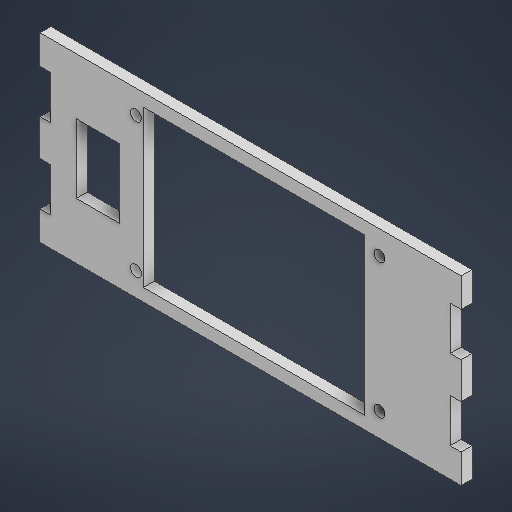
# Autodesk Inventor part: pantallaSoport
Saved by Autodesk Inventor 2026 (Build 300175000, 175)
## iProperties
Created: 2026-04-21
Part Number: pantallaSoport
Material: Generic
Document SubType Name: Modeling
Designer: juana
Density: 1 g/cm^3
Appearance: Default
Author: juana
Autodesk Inventor part; units mm, degrees
ref_plane "YZ Plane" through (0, 0, 0) normal (1, 0, 0) x (0, 1, 0)
ref_plane "XZ Plane" through (0, 0, 0) normal (0, 1, 0) x (-1, 0, 0)
ref_plane "XY Plane" through (0, 0, 0) normal (0, 0, 1) x (1, 0, 0)
sketch "Sketch1" plane through (0, 0, 0) normal (0, 0, 1) x (1, 0, 0)
  line L0 (0, 0) -> (116, 0)
  line L1 (116, 0) -> (116, 50)
  line L2 (116, 50) -> (0, 50)
  line L3 (0, 50) -> (0, 0)
  line L4 (0, 50) -> (3, 50)
  line L5 (3, 50) -> (3, 46.5)
  line L6 (3, 46.5) -> (0, 46.5)
  line L7 (0, 46.5) -> (0, 50)
  line L8 (0, 0) -> (3, 0)
  line L9 (3, 0) -> (3, 3.5)
  line L10 (3, 3.5) -> (0, 3.5)
  line L11 (0, 3.5) -> (0, 0)
  line L12 (58, 0) -> (58, 50) construction
  line L13 (113, 50) -> (113, 46.5)
  line L14 (113, 46.5) -> (116, 46.5)
  line L15 (113, 0) -> (113, 3.5)
  line L16 (113, 3.5) -> (116, 3.5)
  line L17 (19.5, 46.5) -> (96.5, 46.5) construction
  line L18 (96.5, 46.5) -> (96.5, 3.5) construction
  line L19 (96.5, 3.5) -> (19.5, 3.5) construction
  line L20 (19.5, 3.5) -> (19.5, 46.5) construction
  line L21 (28.5, 46.5) -> (89.5, 46.5)
  line L22 (89.5, 46.5) -> (89.5, 3.5)
  line L23 (89.5, 3.5) -> (28.5, 3.5)
  line L24 (28.5, 3.5) -> (28.5, 46.5)
  line L25 (3, 0) -> (0, 0)
  line L26 (0, 0) -> (0, 8)
  line L27 (0, 8) -> (3, 8)
  line L28 (3, 8) -> (3, 0)
  line L29 (0, 50) -> (3, 50)
  line L30 (3, 50) -> (3, 42)
  line L31 (3, 42) -> (0, 42)
  line L32 (0, 42) -> (0, 50)
  line L33 (0, 42) -> (3, 42)
  line L34 (3, 42) -> (3, 30)
  line L35 (3, 30) -> (0, 30)
  line L36 (0, 30) -> (0, 42)
  line L37 (3, 8) -> (0, 8)
  line L38 (0, 8) -> (0, 20)
  line L39 (0, 20) -> (3, 20)
  line L40 (3, 20) -> (3, 8)
  line L41 (116, 8) -> (113, 8)
  line L42 (113, 42) -> (116, 42)
  line L43 (113, 42) -> (113, 30)
  line L44 (113, 30) -> (116, 30)
  line L45 (116, 20) -> (113, 20)
  line L46 (113, 20) -> (113, 8)
  point P0 (1.5, 25)
  point P1 (0, 25)
  point P2 (1.5, 3.5)
  point P3 (19.5, 25)
  point P4 (58, 46.5)
  point P5 (1.5, 46.5)
  point P6 (94.5, 5.5)
  point P7 (94.5, 44.5)
  point P8 (26, 44.5)
  point P9 (26, 5.5)
  point P10 (0, 46.5)
  point P11 (0, 3.5)
  dimension "d0" = 116
  dimension "d1" = 50
  dimension "d2" = 3
  dimension "d4" = 21.5
  dimension "d5" = 21.5
  dimension "d6" = 77
  dimension "d7" = 61
  dimension "d8" = 9
  dimension "d9" = 2
  dimension "d10" = 2
  dimension "d11" = 2
  dimension "d12" = 6.5
  dimension "d13" = 2
  dimension "d34" = 8
  dimension "d35" = 8
  dimension "d36" = 12
  dimension "d37" = 12
  constraints: 94 end point, 18 parallel, 15 symmetric about line, 9 horizontal, 9 perpendicular, 7 midpoint, 7 vertical alignment, 6 horizontal alignment, 2 point on line
  measures "d0" distance of L1.end L2.end
  measures "d1" distance of L0.end L1.end
  measures "d2" distance of L5.end L6.end
  measures "d4" distance from line of L10 point (1.5, 25)
  measures "d5" distance from line of L6 point (1.5, 25)
  measures "d6" distance of L17.start L17.end
  measures "d7" distance of L21.start L21.end
  measures "d8" distance between parallel lines of L20 L24
  measures "d9" distance from line of L19 point (94.5, 5.5)
  measures "d10" distance from line of L17 point (94.5, 44.5)
  measures "d11" distance from line of L18 point (94.5, 44.5)
  measures "d12" distance from line of L20 point (26, 44.5)
  measures "d13" distance from line of L19 point (26, 5.5)
  measures "d34" distance of L27.end L8.end
  measures "d35" distance of L29.end L30.end
  measures "d36" distance of L33.end L34.end
  measures "d37" distance of L39.end L27.end
extrude "Extrusion1" add sketch "Sketch1" along normal blind 3 contours L3 L10 L9 L0 | L9 L28 L40 L39 L3 L35 L34 L30 L5 L2 L13 L14 L1 L42 L43 L44 L45 L46 L41 L16 L15 L0 | L3 L27 L28 L10 | L15 L16 L1 L0 | L3 L6 L30 L31 | L3 L2 L5 L6 | L14 L13 L2 L1
sketch "Sketch2" plane through (0, 0, 3) normal (0, 0, 1) x (1, 0, 0)
  line L0 (28.5, 46.5) -> (89.5, 46.5) projected
  line L1 (19.5, 46.5) -> (96.5, 46.5)
  line L2 (96.5, 46.5) -> (96.5, 3.5)
  line L3 (96.5, 3.5) -> (19.5, 3.5)
  line L4 (19.5, 3.5) -> (19.5, 46.5)
  line L5 (116, 50) -> (0, 50) projected
  line L6 (0, 8) -> (0, 0) projected
  point P0 (26.42, 43.5)
  point P1 (26.42, 6.5)
  point P2 (58, 46.5)
  point P3 (58, 50)
  point P4 (113, 50)
  point P5 (3, 50)
  point P6 (19.5, 25)
  point P7 (0, 25)
  point P8 (0, 46.5)
  point P9 (0, 3.5)
  point P10 (93.5, 43.5)
  point P11 (93.5, 6.5)
  dimension "d17" = 77
  dimension "d18" = 3
  dimension "d19" = 3
  dimension "d20" = 3
  dimension "d28" = 6.92
  constraints: 8 end point, 3 horizontal alignment, 3 midpoint, 3 vertical alignment, 2 parallel, 2 point on line, 1 horizontal, 1 perpendicular
  measures "d17" distance between parallel lines of L2 L4
  measures "d18" distance from line of L1 point (93.5, 43.5)
  measures "d19" distance from line of L3 point (93.5, 6.5)
  measures "d20" distance from line of L2 point (93.5, 6.5)
  measures "d28" distance from line of L4 point (26.42, 6.5)
hole "Hole1" at (26.42, 43.5, 3) at (26.42, 6.5, 3) at (93.5, 6.5, 3) at (93.5, 43.5, 3) direction (0, 0, -1) diameter 3 end through all
sketch "Sketch3" plane through (0, 0, 3) normal (0, 0, 1) x (1, 0, 0)
  line L0 (10, 34.5) -> (22, 34.5)
  line L1 (22, 34.5) -> (22, 15.5)
  line L2 (22, 15.5) -> (10, 15.5)
  line L3 (10, 15.5) -> (10, 34.5)
  line L4 (0, 8) -> (0, 0) construction
  point P0 (10, 25)
  point P1 (0, 25)
  point P2 (0, 46.5)
  point P3 (0, 3.5)
  dimension "d29" = 19
  dimension "d30" = 12
  dimension "d31" = 10
  constraints: 8 end point, 2 parallel, 1 horizontal, 1 horizontal alignment, 1 midpoint, 1 perpendicular, 1 point on line
  measures "d29" distance of L2.end L0.start
  measures "d30" distance of L1.end L2.end
  measures "d31" distance between parallel lines of L4 L3
extrude "Extrusion2" cut sketch "Sketch3" against normal blind 10
body "Solid1"
